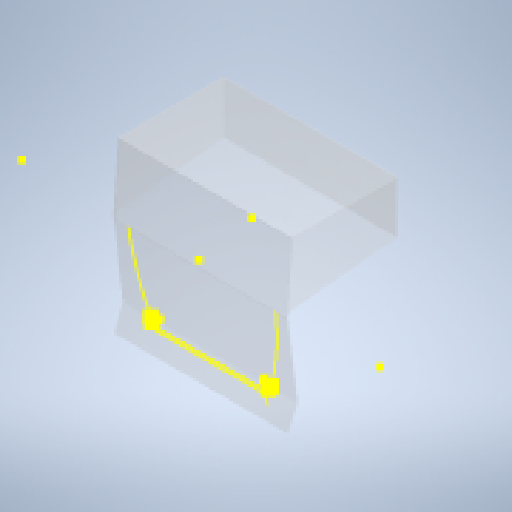
# Autodesk Inventor part: SigmaxxEnclosure
Saved by Autodesk Inventor 2023 (Build 270158000, 158)
## iProperties
Created: 2024-04-02
Part Number: SigmaxxEnclosure
Material: Generic
Document SubType Name: Modeling
Designer: incep
Density: 1 g/cm^3
Appearance: Polycarbonate - Clear
Author: incep
Autodesk Inventor part; units mm, degrees
ref_plane "YZ Plane" through (0, 0, 0) normal (1, 0, 0) x (0, 1, 0)
ref_plane "XZ Plane" through (0, 0, 0) normal (0, 1, 0) x (-1, 0, 0)
ref_plane "XY Plane" through (0, 0, 0) normal (0, 0, 1) x (1, 0, 0)
sketch "Sketch1" plane through (0, 0, 0) normal (0, 1, 0) x (-1, 0, 0)
  line L0 (334.7, -202.665) -> (-334.7, -202.665)
  line L1 (-334.7, -202.665) -> (-334.7, 202.665)
  line L2 (-334.7, 202.665) -> (334.7, 202.665)
  line L3 (334.7, 202.665) -> (334.7, -202.665)
  line L4 (337.7, -202.665) -> (-337.7, -202.665) construction
  line L5 (-337.7, -202.665) -> (-337.7, 202.665) construction
  line L6 (-337.7, 202.665) -> (337.7, 202.665) construction
  line L7 (337.7, 202.665) -> (337.7, -202.665) construction
  line L8 (-331.7, 199.665) -> (-331.7, -199.665)
  line L9 (-331.7, -199.665) -> (331.7, -199.665)
  line L10 (331.7, -199.665) -> (331.7, 199.665)
  line L11 (331.7, 199.665) -> (-331.7, 199.665)
  line L12 (331.7, 199.665) -> (331.7, 202.665)
  line L13 (-331.7, 199.665) -> (-331.7, 202.665)
  line L14 (331.7, -199.665) -> (331.7, -202.665)
  line L15 (-331.7, -199.665) -> (-331.7, -202.665)
  point P0 (0, 0)
  point P1 (-334.7, 0)
  point P2 (0, -202.665)
  point P3 (0, -202.665)
  point P4 (-337.7, 0)
  point P5 (331.7, 202.665)
  point P6 (331.7, -202.665)
  point P7 (-331.7, -202.665)
  dimension "d0" = 675.4
  dimension "d1" = 405.33
  dimension "d2" = 3
  dimension "d3" = 3
  constraints: 32 end point, 6 parallel, 6 perpendicular, 4 midpoint, 4 point on line, 2 horizontal, 2 horizontal alignment, 2 vertical alignment, 1 collinear, 1 vertical, 3 other
  measures "d0" distance of L4.start L4.end
  measures "d1" distance of L6.end L4.start
  measures "d2" distance between parallel lines of L5 L1
  measures "d3" distance between parallel lines of L1 L8
extrude "Extrusion1" add sketch "Sketch1" along normal blind 200 contours L0 L14 L10 L12 L2 L3
extrude "Extrusion2" add sketch "Sketch1" along normal blind 200 separate body contours L0 L15 L9 L14
sketch "Sketch2" plane through (-334.7, 0, -202.665) normal (-1, 0, 0) x (0, 0, 1)
  line L0 (405.33, 0) -> (0, 0) projected
  line L1 (0, 0) -> (405.33, -39.3)
  line L2 (405.33, 0) -> (405.33, -39.3) construction
  line L3 (405.33, 0) -> (405.33, 200) projected
  arc A0 (421.4573, -59.4215) -> (405.33, -39.3) centre (403.5929, -57.216) ccw
  line L4 (421.4573, -59.4215) -> (413.7818, -121.5922) construction
  line L5 (421.4573, -59.4215) -> (424.4347, -59.7891)
  line L6 (405.33, 200) -> (424.4347, -59.7891)
  point P0 (202.665, 0)
  dimension "d8" = 39.3
  dimension "d9" = 18
  dimension "d10" = 88.5
  dimension "d12" = 3
  constraints: 10 end point, 2 point on circle, 2 tangent, 1 centre point, 1 collinear, 1 line through centre, 1 vertical, 1 vertical alignment
  measures "d8" distance of L0.start L1.end
  measures "d9" radius of A0
  measures "d10" angle of L4 L1
  measures "d12" distance of L4.start L5.end
extrude "Extrusion3" add sketch "Sketch2" against normal up to surface (3 mm away) bodies 1
mirror "Mirror1" about plane through (0, 0, 0) normal (1, 0, 0) of "Extrusion3", "Extrusion1" bodies 1
sketch "Sketch4" plane through (-334.7, 0, -202.665) normal (-1, 0, 0) x (0, 0, 1)
  line L0 (0, 0) -> (405.33, -39.3) projected
  arc A0 (421.4573, -59.4215) -> (405.33, -39.3) centre (403.5929, -57.216) ccw projected
  line L1 (421.4573, -59.4215) -> (424.4347, -59.7891) projected
  line L2 (424.4347, -59.7891) -> (405.33, 200) projected
  line L3 (0, 200) -> (405.33, 200) projected
  line L4 (0, 0) -> (0, 200) projected
  line L5 (424.4347, -59.7891) -> (405.33, 200) projected
  line L6 (405.33, 200) -> (408.33, 200.2206)
  line L7 (408.33, 200.2206) -> (427.4266, -59.569)
  line L8 (424.4347, -59.7891) -> (427.4266, -59.569)
  point P0 (202.665, 0)
  dimension "d15" = 90
  dimension "d16" = 3
  dimension "d17" = 90
  dimension "d19" = 3
  constraints: 6 end point
  measures "d15" angle of L6 L2
  measures "d16" horizontal distance of L2.end L6.end
  measures "d17" angle of L2 L8
  measures "d19" distance of L1.end L7.end
extrude "Extrusion4" add sketch "Sketch4" against normal up to surface (669.4 mm away) separate body contours L6 L7 L8 L2
sketch "Sketch5" plane through (0, 200, 0) normal (0, 1, 0) x (1, 0, 0)
  line L0 (-334.7, 202.665) -> (-334.7, -202.665) projected
  line L1 (334.7, -218.9279) -> (334.7, -202.665) projected
  line L2 (-334.7, 202.665) -> (334.7, 202.665)
  line L3 (334.7, 202.665) -> (334.7, -205.7675)
  line L4 (334.7, -205.7675) -> (-334.7, -205.7675)
  line L5 (-334.7, -205.7675) -> (-334.7, 202.665)
  point P0 (0, 0)
  point P1 (334.7, -218.7923)
  constraints: 8 end point, 2 parallel, 1 horizontal, 1 perpendicular, 1 point on line
extrude "Extrusion5" add sketch "Sketch5" against normal blind 3 separate body
sketch "Sketch6" plane through (-334.7, 0, -202.665) normal (-1, 0, 0) x (0, 0, 1)
  arc A0 (421.4573, -59.4215) -> (405.33, -39.3) centre (403.5929, -57.216) ccw projected
  line L0 (421.4573, -59.4215) -> (385.3424, -351.9506)
  arc A1 (421.4573, -59.4215) -> (405.33, -39.3) centre (403.5929, -57.216) ccw projected
  arc A2 (385.3424, -351.9506) -> (387.6008, -367.5802) centre (415.1163, -355.6264) ccw
  line L1 (387.6008, -367.5802) -> (421.0197, -444.5046)
  line L2 (424.4347, -59.7891) -> (388.3198, -352.3182)
  arc A3 (388.3198, -352.3182) -> (390.3523, -366.3849) centre (415.1163, -355.6264) ccw
  line L3 (390.3523, -366.3849) -> (423.7713, -443.3092)
  line L4 (421.4573, -59.4215) -> (424.4347, -59.7891)
  line L5 (421.0197, -444.5046) -> (423.7713, -443.3092)
  point P0 (202.665, 0)
  dimension "d24" = 294.75
  dimension "d25" = 30
  dimension "d26" = 149.48
  dimension "d27" = 83.87
  dimension "d28" = 3
  constraints: 12 end point, 4 point on circle, 3 tangent, 2 centre point, 1 perpendicular, 2 other
  measures "d24" distance of L0.start L0.end
  measures "d25" radius of A2
  measures "d26" angle of L0 L1
  measures "d27" distance of L1.start L1.end
  measures "d28" distance between parallel lines of L0 L2
extrude "Extrusion6" add sketch "Sketch6" against normal up to surface (669.4 mm away) separate body
sketch "Sketch7" plane through (-334.7, -59.7891, 221.7697) normal (0, -0.1225, 0.9925) x (1, 0, 0)
  ellipse E0 centre (1026.9236, 18.0035) end of major axis (1999.1461, 18.0035) minor radius 972.2223 (54.8677, 0.0035) -> (106.3768, -294.7427) ccw projected
  spline S0 degree 3 poles (109, -302.3594) (108.5627, -301.1176) (108.1258, -299.8562) (107.2511, -297.3094) (106.8142, -296.0268) (106.3768, -294.7427) knots -0.813889 -0.813889 -0.813889 -0.813889 -0.406945 -0.406945 0 0 0 0 projected
  spline S1 degree 3 poles (112.888, -309.9746) (112.3974, -309.2284) (111.9723, -308.5468) (111.6126, -307.9425) (111.4327, -307.6404) (111.2692, -307.3574) (111.1221, -307.0949) (111.0485, -306.9636) (110.979, -306.8374) (110.9136, -306.7164) (110.8809, -306.6559) (110.8493, -306.5967) (110.8186, -306.5388) (110.8033, -306.5098) (110.7882, -306.4812) (110.7734, -306.4529) (110.766, -306.4387) (110.7586, -306.4247) (110.7514, -306.4107) (110.7441, -306.3967) (110.7375, -306.384) (110.7297, -306.369) (110.2337, -305.4107) (109.6571, -304.0867) (109, -302.3594) knots 0 0 0 0 0.25 0.25 0.25 0.375 0.375 0.375 0.4375 0.4375 0.4375 0.46875 0.46875 0.46875 0.484375 0.484375 0.484375 0.492187 0.492187 0.492187 0.5 0.5 0.5 1 1 1 1 projected
  ellipse E1 centre (138.7441, -291.9833) end of major axis (170.2478, -291.9833) minor radius 31.4913 (112.888, -309.9746) -> (138.7441, -323.4747) ccw projected
  line L0 (138.7441, -323.4747) -> (536.6559, -323.4747) projected
  ellipse E2 centre (138.7441, -291.9833) end of major axis (170.2478, -291.9833) minor radius 31.4913 (112.888, -309.9746) -> (138.7441, -323.4747) ccw projected
  line L1 (138.7441, -323.4747) -> (536.6559, -323.4747) projected
  line L2 (543.4, -374.2271) -> (543.4, -316.9082) projected
  ellipse E3 centre (-351.5236, 18.0035) end of major axis (620.6989, 18.0035) minor radius 972.2223 (569.0232, -294.7427) -> (620.5323, 0.0035) ccw projected
  spline S2 degree 3 poles (569.0232, -294.7427) (568.5858, -296.0268) (568.1489, -297.3094) (567.2742, -299.8562) (566.8373, -301.1176) (566.4, -302.3594) knots -0.813889 -0.813889 -0.813889 -0.813889 -0.406945 -0.406945 0 0 0 0 projected
  ellipse E4 centre (-351.5236, 18.0035) end of major axis (620.6989, 18.0035) minor radius 972.2223 (569.0232, -294.7427) -> (620.5323, 0.0035) ccw projected
  spline S3 degree 3 poles (566.4, -302.3594) (566.0715, -303.2229) (565.7631, -303.9859) (565.3307, -304.986) (565.1916, -305.2952) (564.9904, -305.724) (564.9246, -305.8611) (564.8278, -306.058) (564.7799, -306.1543) (564.7248, -306.2629) (564.7014, -306.3087) (564.6858, -306.339) (564.6774, -306.3552) (564.4415, -306.811) (564.1473, -307.338) (563.4278, -308.5466) (563.0027, -309.2282) (562.512, -309.9746) knots 0 0 0 0 0.25 0.25 0.375 0.375 0.4375 0.4375 0.46875 0.484375 0.492187 0.492187 0.5 0.5 0.75 0.75 1 1 1 1 projected
  ellipse E5 centre (536.6559, -291.9833) end of major axis (568.1595, -291.9833) minor radius 31.4913 (536.6559, -323.4747) -> (562.512, -309.9746) ccw projected
  point P0 (334.7, 32.1657)
  constraints: 6 other
sketch "Sketch8" plane through (-334.7, -366.3849, 187.6873) normal (0, 0.3985, 0.9172) x (1, 0, 0)
  line L0 (138.7441, -15.6403) -> (536.6559, -15.6403) projected
  ellipse E0 centre (138.7441, 20.9297) end of major axis (138.7441, 57.4996) minor radius 31.5036 (112.888, 0.037) -> (138.7441, -15.6403) ccw projected
  ellipse E1 centre (536.6559, 20.9297) end of major axis (536.6559, -15.6403) minor radius 31.5036 (536.6559, -15.6403) -> (562.512, 0.037) ccw projected
  spline S0 degree 3 poles (566.4, 8.211) (566.0715, 7.3517) (565.7631, 6.5717) (565.3307, 5.5321) (565.1916, 5.2072) (564.9904, 4.7533) (564.9246, 4.6076) (564.8278, 4.3974) (564.7799, 4.2944) (564.7248, 4.1779) (564.7014, 4.1288) (564.6858, 4.0962) (564.6774, 4.0788) (564.4415, 3.5887) (564.1473, 3.0158) (563.4278, 1.6734) (563.0027, 0.9037) (562.512, 0.037) knots 0 0 0 0 0.25 0.25 0.375 0.375 0.4375 0.4375 0.46875 0.484375 0.492187 0.492187 0.5 0.5 0.75 0.75 1 1 1 1 projected
  spline S1 degree 3 poles (112.888, 0.037) (112.3974, 0.9036) (111.9723, 1.6732) (111.6126, 2.3444) (111.4327, 2.68) (111.2692, 2.991) (111.1221, 3.2776) (111.0485, 3.4209) (110.979, 3.558) (110.9136, 3.6891) (110.8809, 3.7546) (110.8493, 3.8186) (110.8186, 3.8811) (110.8033, 3.9123) (110.7882, 3.9432) (110.7734, 3.9736) (110.766, 3.9889) (110.7586, 4.004) (110.7514, 4.0191) (110.7441, 4.0341) (110.7375, 4.0478) (110.7297, 4.0639) (110.2337, 5.0945) (109.6571, 6.4921) (109, 8.211) knots 0 0 0 0 0.25 0.25 0.25 0.375 0.375 0.375 0.4375 0.4375 0.4375 0.46875 0.46875 0.46875 0.484375 0.484375 0.484375 0.492187 0.492187 0.492187 0.5 0.5 0.5 1 1 1 1 projected
  point P0 (334.7, 410.8289)
  constraints: 2 other
